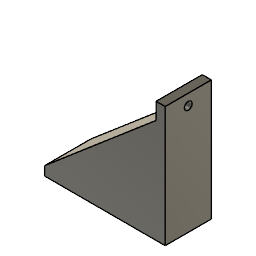
L hold (Autodesk Fusion 360 design; units mm, degrees)
part number: 2026-03-30-19-16-17-509
Autodesk Fusion 360 part; units mm, degrees
sketch "Sketch1" plane through (0, 0, 0) normal (0, 0, 1) x (1, 0, 0)
  line L0 (0, 0) -> (5.7785, 0)
  line L1 (5.7785, 0) -> (5.7785, 29.21)
  line L2 (5.7785, 29.21) -> (0, 29.21)
  line L3 (0, 29.21) -> (0, 0)
  line L4 (0, 29.21) -> (76.2, 29.21)
  line L5 (76.2, 29.21) -> (76.2, 0)
  line L6 (76.2, 0) -> (0, 0)
  line L7 (0, 0) -> (0, 29.21)
  circle A0 centre (69.3074, 14.605) radius 2.4447
  line L8 (69.3074, 14.605) -> (69.3074, 29.21) construction
  line L9 (69.3074, 14.605) -> (69.3074, 0) construction
  dimension "d1" = 29.21
  dimension "d2" = 5.7785
  dimension "d3" = 29.21
  dimension "d4" = 76.2
  dimension "d11" = 4.8895
  constraint horizontal L0
  constraint vertical L1
  constraint horizontal L2
  constraint vertical L3
  constraint coincident L0.start L3.end
  constraint horizontal L4
  constraint vertical L5
  constraint horizontal L6
  constraint vertical L7
  constraint coincident A0.centre L8.start
  constraint coincident L4 L8.end
  constraint perpendicular L4 L8
  constraint coincident L6 L9.end
  constraint perpendicular L6 L9
  constraint equal L8 L9
  measures "d1" distance of L0.start L2.end
  measures "d2" distance of L0.start L0.end
  measures "d3" distance of L2.end L0.start
  measures "d4" distance of L5.end L0.start
  measures "d11" diameter of A0
extrude "Extrude1" add sketch "Sketch1" along normal blind 76.2 contours L0 L1 L2 L3 L4 L6 L7
extrude "Extrude2" add sketch "Sketch1" along normal blind 5.7785 contours L1 L4 L5 L6 | A0
sketch "Sketch2" plane through (0, 0, 0) normal (0, 1, 0) x (1, 0, 0)
  line L0 (5.7785, -76.2) -> (66.6409, -4.6543)
  line L1 (66.6409, -4.6543) -> (5.7785, -4.6543)
  line L2 (5.7785, -4.6543) -> (5.7785, -76.2)
  line L3 (0, -76.2) -> (5.7785, -76.2)
  constraint horizontal L1
  constraint perpendicular L1 L2
  constraint coincident L0.start L2.end
extrude "Extrude3" add sketch "Sketch2" along normal blind 29.21
extrude "Extrude4" cut sketch "Sketch1" along normal blind 6.2865 contours A0
sketch "Sketch4" plane through (0, 0, 0) normal (1, 0, 0) x (0, 1, 0)
  circle A0 centre (24.1427, 20.1486) radius 2.4447
  line L0 (29.21, 0) -> (0, 0)
  circle A1 centre (24.1427, 20.1486) radius 3.9817
  dimension "d15" = 4.8895
  dimension "d16" = 20.1485
  constraint concentric A0 A1
  measures "d15" diameter of A0
  measures "d16" distance of A0.centre L0
extrude "Extrude5" cut sketch "Sketch4" along normal blind 55 contours A0
sketch "Sketch5" plane through (0, 0, 0) normal (-1, 0, 0) x (0, -1, 0)
  circle A0 centre (-24.1427, 20.1486) radius 2.4447
  line L0 (-29.21, 0) -> (0, 0)
  line L1 (0, 0) -> (0, 76.2)
  line L2 (0, 76.2) -> (-29.21, 76.2)
  line L3 (-29.21, 76.2) -> (-29.21, 0)
  line L4 (-27.4447, 42.0226) -> (-20.8407, 42.0226)
  line L5 (-20.8407, 42.0226) -> (-20.8407, 35.4186)
  line L6 (-20.8407, 35.4186) -> (-27.4447, 35.4186)
  line L7 (-27.4447, 35.4186) -> (-27.4447, 42.0226)
  line L8 (-27.4447, 38.7206) -> (-20.8407, 38.7206) construction
  line L9 (-24.1427, 42.0226) -> (-24.1427, 35.4186) construction
  point P0 (-24.1427, 38.7206)
  point P1 (-14.605, 0)
  dimension "d19" = 39.878
  dimension "d20" = 6.604
  constraint horizontal L4
  constraint vertical L5
  constraint horizontal L6
  constraint vertical L7
  constraint midpoint L7 L8.start
  constraint midpoint L5 L8.end
  constraint midpoint L4 L9.start
  constraint midpoint L6 L9.end
  constraint midpoint L8 P0
  constraint equal L5 L6
  measures "d19" distance of P0 P1
  measures "d20" distance of L4.start L4.end
extrude "Extrude6" cut sketch "Sketch5" against normal blind 5.7912 contours L4 L5 L6 L7
extrude "Extrude7" cut sketch "Sketch4" along normal blind 55 from surface at 5.08 contours A0 | A1
move_body "Move1" bodies 1 to x (0, 0, 1) y (0, 1, 0) z (-1, 0, 0) at (25.2286, 0, 0.0685)
